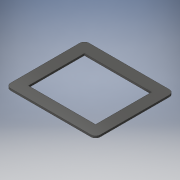
# Autodesk Inventor part: Border
Saved by Autodesk Inventor 2016 (Build 200138000, 138)
## iProperties
Created: 2015-08-29
Part Number: Border
Material: Rubber
Document SubType Name: Modeling
Designer: Pranav
Density: 0.93 g/cm^3
Appearance: Diamond plate - Dark Gray
Author: Pranav
Autodesk Inventor part; units mm, degrees
ref_plane "YZ Plane" through (0, 0, 0) normal (1, 0, 0) x (0, 1, 0)
ref_plane "XZ Plane" through (0, 0, 0) normal (0, 1, 0) x (-1, 0, 0)
ref_plane "XY Plane" through (0, 0, 0) normal (0, 0, 1) x (1, 0, 0)
sketch "Sketch1" plane through (0, 0, 0) normal (0, 1, 0) x (-1, 0, 0)
  line L0 (0, 0) -> (1828.8, 0)
  line L1 (1828.8, 0) -> (1828.8, -1524)
  line L2 (1828.8, -1524) -> (0, -1524)
  line L3 (0, -1524) -> (0, 0)
  line L4 (2133.6, 304.8) -> (-304.8, 304.8)
  line L5 (-304.8, 304.8) -> (-304.8, -1828.8)
  line L6 (-304.8, -1828.8) -> (2133.6, -1828.8)
  line L7 (2133.6, -1828.8) -> (2133.6, 304.8)
  dimension "d0" = 1828.8
  dimension "d1" = 1524
  dimension "d2" = 304.8
  dimension "d3" = 304.8
  dimension "d4" = 304.8
  dimension "d5" = 304.8
  constraints: 16 end point, 4 parallel, 2 horizontal, 2 perpendicular
  measures "d0" distance of L1.end L2.end
  measures "d1" distance of L0.end L1.end
  measures "d2" distance between parallel lines of L6 L2
  measures "d3" distance between parallel lines of L0 L4
  measures "d4" distance between parallel lines of L5 L3
  measures "d5" distance between parallel lines of L1 L7
extrude "Extrusion1" add sketch "Sketch1" along normal blind 50.8
fillet "Fillet1" radius 127 1 edges at (304.8, 25.4, 304.8)
fillet "Fillet2" radius 127 1 edges at (304.8, 25.4, -1828.8)
fillet "Fillet3" radius 127 1 edges at (-2133.6, 25.4, -1828.8)
fillet "Fillet4" radius 127 1 edges at (-2133.6, 25.4, 304.8)
body "Solid1"
